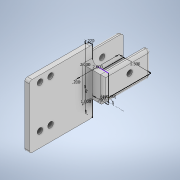
# Autodesk Inventor part: USAXS mount to 1 in 8020
Saved by Autodesk Inventor 2020 (Build 240168000, 168)
## iProperties
Created: 2022-02-15
Part Number: USAXS mount to 1 in 8020
Material: Generic
Document SubType Name: Modeling
Designer: Beaucage
Density: 1 g/cm^3
Appearance: Default
Author: Beaucage
Autodesk Inventor part; units mm, degrees
ref_plane "YZ Plane" through (0, 0, 0) normal (1, 0, 0) x (0, 1, 0)
ref_plane "XZ Plane" through (0, 0, 0) normal (0, 1, 0) x (-1, 0, 0)
ref_plane "XY Plane" through (0, 0, 0) normal (0, 0, 1) x (1, 0, 0)
sketch "Sketch1" plane through (0, 0, 0) normal (0, 1, 0) x (-1, 0, 0)
  line L0 (0, 0) -> (38.1, 0)
  line L1 (38.1, 0) -> (38.1, -50.8)
  line L2 (38.1, -50.8) -> (0, -50.8)
  line L3 (0, -50.8) -> (0, 0)
  line L4 (38.1, -50.8) -> (33.02, -50.8)
  line L5 (33.02, -50.8) -> (33.02, 0)
  line L6 (33.02, 0) -> (38.1, 0)
  line L7 (38.1, 0) -> (38.1, -50.8)
  line L8 (0, -50.8) -> (5.08, -50.8)
  line L9 (5.08, -50.8) -> (5.08, 0)
  line L10 (5.08, 0) -> (0, 0)
  line L11 (0, 0) -> (0, -50.8)
  dimension "d0" = 38.1
  dimension "d1" = 50.8
  dimension "d2" = 5.08
  dimension "d3" = 5.08
  constraints: 24 end point, 6 parallel, 3 horizontal, 3 perpendicular, 2 point on line
  measures "d0" distance of L1.end L2.end
  measures "d1" distance of L0.end L1.end
  measures "d2" distance of L5.end L6.end
  measures "d3" distance of L10.end L9.end
extrude "Extrusion1" add sketch "Sketch1" along normal blind 25.4 contours L0 L9 L2 L3 | L0 L1 L2 L5
extrude "Extrusion2" add sketch "Sketch1" against normal blind 5.08
sketch "Sketch2" plane through (0, 25.4, 0) normal (1, 0, 0) x (0, 0, -1)
  line L0 (50.8, 0) -> (0, 0) projected
  line L1 (25.4, 0) -> (25.4, -12.7)
  point P0 (0, -25.4)
  dimension "d8" = 12.7
  constraints: 2 end point, 1 midpoint, 1 vertical
  measures "d8" distance of L1.start L1.end
hole "Hole1" at (0, 12.7, -25.4) direction (-1, 0, 0) diameter 6.7564 end through all clearance for "Socket Head Cap Screw" size "1/4" standard "Ansi Unified Screw Threads"
sketch "Sketch3" plane through (-5.08, 25.4, 0) normal (0, 0, 1) x (1, 0, 0)
  line L0 (5.08, -30.48) -> (5.08, 0) projected
  line L1 (5.08, -30.48) -> (-13.97, -30.48)
  line L2 (5.08, -30.48) -> (24.13, -30.48) construction
  line L3 (-13.97, -30.48) -> (-19.558, -30.48)
  line L4 (-19.558, -30.48) -> (-19.558, 20.32)
  line L5 (-19.558, 20.32) -> (-13.97, 20.32)
  line L6 (-13.97, 20.32) -> (-13.97, -30.48)
  line L7 (-33.02, -30.48) -> (-33.02, 0) projected
  line L8 (-33.02, 0) -> (-19.558, 0)
  line L9 (-19.558, 0) -> (-19.558, -30.48)
  line L10 (-19.558, -30.48) -> (-33.02, -30.48)
  line L11 (-33.02, -30.48) -> (-33.02, 0)
  line L12 (-13.97, -30.48) -> (-19.558, -30.48)
  line L13 (-19.558, -30.48) -> (-19.558, -55.88)
  line L14 (-19.558, -55.88) -> (-13.97, -55.88)
  line L15 (-13.97, -55.88) -> (-13.97, -30.48)
  line L16 (5.08, -30.48) -> (-13.97, -30.48)
  line L17 (-13.97, -30.48) -> (-13.97, 0)
  line L18 (-13.97, 0) -> (5.08, 0)
  line L19 (5.08, 0) -> (5.08, -30.48)
  point P0 (5.08, -25.4)
  dimension "d16" = 19.05
  dimension "d17" = 180
  dimension "d18" = 5.588
  dimension "d19" = 50.8
  dimension "d20" = 25.4
  constraints: 36 end point, 8 parallel, 6 horizontal, 4 perpendicular, 2 point on line, 1 collinear
  measures "d16" distance of L0.start L1.end
  measures "d17" angle of L1 L2
  measures "d18" distance of L4.end L5.end
  measures "d19" distance of L3.end L4.end
  measures "d20" distance of L13.end L12.end
extrude "Extrusion3" add sketch "Sketch3" along normal blind 6.35 contours L1 L6 L18 L0 | L10 L7 L8 L4
extrude "Extrusion4" add sketch "Sketch3" along normal blind 76.2 contours L15 L14 L13 L3 | L3 L4 L5 L6
sketch "Sketch4" plane through (-19.05, -30.48, 0) normal (1, 0, 0) x (0, 0, -1)
  line L0 (50.8, 55.88) -> (0, 55.88) projected
  line L1 (0, 55.88) -> (-76.2, 55.88)
  line L2 (-76.2, 76.2) -> (-76.2, 0) projected
  line L3 (-76.2, 55.88) -> (-63.5, 55.88)
  line L4 (-76.2, 55.88) -> (-63.5, 55.88) construction
  line L5 (-63.5, 55.88) -> (-50.8, 55.88)
  line L6 (-50.8, 55.88) -> (-50.8, 68.58)
  line L7 (-63.5, 55.88) -> (-63.5, 68.58)
  line L8 (-50.8, 68.58) -> (-50.8, 17.78)
  line L9 (-63.5, 68.58) -> (-63.5, 17.78)
  point P0 (0, 30.48)
  dimension "d25" = 12.7
  dimension "d26" = 0
  dimension "d27" = 12.7
  dimension "d28" = 12.7
  dimension "d29" = 50.8
  constraints: 16 end point, 3 vertical, 2 collinear, 2 horizontal, 2 point on line, 1 perpendicular
  measures "d25" distance of L1.end L3.end
  measures "d26" distance between parallel lines of L3 L4
  measures "d27" distance of L3.end L5.end
  measures "d28" distance of L5.end L6.end
  measures "d29" distance of L6.end L8.end
hole "Hole2" at (-19.05, 38.1, 50.8) at (-19.05, 38.1, 63.5) at (-19.05, -12.7, 63.5) at (-19.05, -12.7, 50.8) direction (-1, 0, 0) diameter 6.7564 end through all clearance for "Socket Head Cap Screw" size "1/4" standard "Ansi Unified Screw Threads"
fillet "Fillet1" radius 6.35 6 edges at (-19.05, 10.16, 6.35) (-19.05, -5.08, 3.175) (-19.05, 25.4, 3.175) (-24.638, 25.4, 3.175) (-24.638, 10.16, 6.35) (-24.638, -5.08, 3.175)
fillet "Fillet2" radius 3.175 10 edges at (-38.1, 10.16, 6.35) (-38.1, -5.08, -22.225) (-38.1, 25.4, -22.225) (0, 25.4, -22.225) (0, 10.16, 6.35) (0, -5.08, -22.225) (-21.844, 45.72, 76.2) (-21.844, -30.48, 76.2) (-21.844, 45.72, 0) (-21.844, -30.48, 0)
fillet "Fillet3" radius 6.35 1 edges at (-21.844, -5.08, 0)
fillet "Fillet4" radius 3.175 9 edges at (-37.1701, 24.4701, -50.8) (-33.9725, 25.4, -50.8) (-37.1701, -4.1501, -50.8) (-19.05, -5.08, -50.8) (-0.9299, -4.1501, -50.8) (0, 10.16, -50.8) (-0.9299, 24.4701, -50.8) (-4.1275, 25.4, -50.8) (-38.1, 10.16, -50.8)
body "Solid1"
